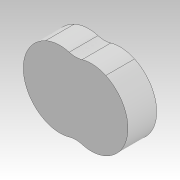
# Autodesk Inventor part: Rotor_NEW
Saved by Autodesk Inventor 2020 (Build 240168000, 168)
## iProperties
Created: 2022-01-30
Part Number: Rotor_NEW
Material: Generic
Document SubType Name: Modeling
Designer: DDeGo
Density: 1 g/cm^3
Appearance: Default
Author: DDeGo
Autodesk Inventor part; units mm, degrees
ref_plane "YZ Plane" through (0, 0, 0) normal (1, 0, 0) x (0, 1, 0)
ref_plane "XZ Plane" through (0, 0, 0) normal (0, 1, 0) x (-1, 0, 0)
ref_plane "XY Plane" through (0, 0, 0) normal (0, 0, 1) x (1, 0, 0)
sketch "Sketch1" plane through (0, 0, 0) normal (0, 0, 1) x (1, 0, 0)
  line L0 (5.3, 0) -> (-5.3, 0) construction
  line L1 (5.3, 14.7) -> (-5.3, 14.7) construction
  arc A0 (20, 0) -> (11.5297, 13.3147) centre (5.3, 0) ccw
  arc A1 (-5.3, 14.7) -> (-11.5297, 13.3147) centre (-5.3, 0) ccw construction
  line L2 (-20, 24.8831) -> (20, 24.8831) construction
  line L3 (20, 24.8831) -> (20, -24.8831) construction
  line L4 (20, -24.8831) -> (-20, -24.8831) construction
  line L5 (-20, -24.8831) -> (-20, 24.8831) construction
  line L6 (0, 0) -> (0, 14.7) construction
  arc A2 (-2.4629, 14.0436) -> (0, 13.7) centre (0, 22.7) ccw
  arc A3 (-2.4629, 14.0436) -> (-11.5297, 13.3147) centre (-6.0204, 1.5398) ccw
  arc A4 (-11.5297, 13.3147) -> (-20, 0) centre (-5.3, 0) ccw
  arc A5 (0, 13.7) -> (2.4629, 14.0436) centre (0, 22.7) ccw
  arc A6 (11.5297, 13.3147) -> (2.4629, 14.0436) centre (6.0204, 1.5398) ccw
  arc A7 (11.5297, 13.3147) -> (5.3, 14.7) centre (5.3, 0) ccw construction
  line L7 (-20, 0) -> (20, 0) construction
  arc A8 (11.5297, -13.3147) -> (20, 0) centre (5.3, 0) ccw
  arc A9 (0, -13.7) -> (-2.4629, -14.0436) centre (0, -22.7) ccw
  arc A10 (-11.5297, -13.3147) -> (-2.4629, -14.0436) centre (-6.0204, -1.5398) ccw
  arc A11 (-20, 0) -> (-11.5297, -13.3147) centre (-5.3, 0) ccw
  arc A12 (2.4629, -14.0436) -> (0, -13.7) centre (0, -22.7) ccw
  arc A13 (2.4629, -14.0436) -> (11.5297, -13.3147) centre (6.0204, -1.5398) ccw
  circle A14 centre (0, 0) radius 2.5
  dimension "d0" = 14.7
  dimension "d1" = 40
  dimension "d2" = 1
  dimension "d3" = 9
  dimension "d4" = 13
  dimension "d5" = 5
  constraints: 28 point on circle, 18 end point, 15 centre point, 12 tangent, 9 symmetric about line, 5 midpoint, 3 point on line, 2 equal radius, 2 horizontal, 2 parallel, 1 coincident, 1 perpendicular, 1 vertical, 6 other
  measures "d0" radius of A1
  measures "d1" distance of L2.start L2.end
  measures "d2" distance from line of L1 A2.end
  measures "d3" radius of A2
  measures "d4" radius of A3
  measures "d5" diameter of A14
extrude "Extrusion1" add sketch "Sketch1" along normal mid plane 11 contours A8 A13 A12 A9 A10 A11 A4 A3 A2 A5 A6 A0 | A14
body "Solid1"
